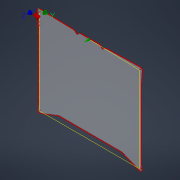
# Autodesk Inventor part: left_plate_02
Saved by Autodesk Inventor 2022 (Build 260153000, 153)
## iProperties
Created: 2025-02-08
Part Number: left_plate_02
Material: ポリカーボネート、クリア
Document SubType Name: Modeling
Designer: gisen
Density: 1.2 g/cm^3
Appearance: ポリカーボネート - クリア
Mass: 702.693 g
Surface Area: 3961.4 cm^2
Volume: 585.578 cm^3
Author: gisen
Autodesk Inventor part; units mm, degrees
ref_plane "YZ Plane" through (0, 0, 0) normal (1, 0, 0) x (0, 1, 0)
ref_plane "XZ Plane" through (0, 0, 0) normal (0, 1, 0) x (-1, 0, 0)
ref_plane "XY Plane" through (0, 0, 0) normal (0, 0, 1) x (1, 0, 0)
sketch "スケッチ1" plane through (0, 0, 0) normal (0, 0, 1) x (1, 0, 0)
  circle A0 centre (-239, 204) radius 2.1 construction
  circle A1 centre (-239, -204) radius 2.1 construction
  circle A2 centre (239, -204) radius 2.1 construction
  circle A3 centre (239, 204) radius 2.1 construction
  circle A4 centre (-61, 204) radius 2.1 construction
  circle A5 centre (61, 204) radius 2.1 construction
  circle A6 centre (-50, -185) radius 2.1 construction
  circle A7 centre (-161.1336, -215) radius 2.1 construction
  circle A8 centre (50, -185) radius 2.1 construction
  circle A9 centre (150, -185) radius 2.1 construction
  circle A10 centre (161.1336, -215) radius 2.1 construction
  circle A11 centre (250, -185) radius 1.6 construction
  circle A12 centre (250, -215) radius 1.6 construction
  line L0 (239, 184) -> (239, -154) construction
  arc A13 (239, 184) -> (219, 204) centre (219, 184) ccw construction
  arc A14 (219, -174) -> (239, -154) centre (219, -154) ccw construction
  line L1 (219, -174) -> (-219, -174) construction
  line L2 (81, 204) -> (219, 204) construction
  line L3 (-239, -154) -> (-239, 184) construction
  arc A15 (-239, -154) -> (-219, -174) centre (-219, -154) ccw construction
  arc A16 (-219, 204) -> (-239, 184) centre (-219, 184) ccw construction
  line L4 (-219, 204) -> (-81, 204) construction
  arc A17 (-66.8579, 198.1421) -> (-55.1421, 198.1421) centre (-61, 204) ccw construction
  arc A18 (-66.8579, 198.1421) -> (-81, 204) centre (-81, 184) ccw construction
  arc A19 (-41, 204) -> (-55.1421, 198.1421) centre (-41, 184) ccw construction
  line L5 (-41, 204) -> (41, 204) construction
  arc A20 (55.1421, 198.1421) -> (41, 204) centre (41, 184) ccw construction
  arc A21 (55.1421, 198.1421) -> (66.8579, 198.1421) centre (61, 204) ccw construction
  arc A22 (81, 204) -> (66.8579, 198.1421) centre (81, 184) ccw construction
  circle A23 centre (-250, -215) radius 2.1 construction
  circle A24 centre (-239, 204) radius 10 construction
  circle A25 centre (-250, 215) radius 1.6 construction
  circle A26 centre (-250, 215) radius 5 construction
  circle A27 centre (-239, -204) radius 10 construction
  circle A28 centre (239, -204) radius 10 construction
  circle A29 centre (239, 204) radius 10 construction
  line L6 (245, -154) -> (245, 184) construction
  arc A30 (245, 184) -> (219, 210) centre (219, 184) ccw construction
  line L7 (219, 210) -> (81, 210) construction
  arc A31 (81, 210) -> (62.6152, 202.3848) centre (81, 184) ccw construction
  arc A32 (59.3848, 202.3848) -> (62.6152, 202.3848) centre (61, 204) ccw construction
  arc A33 (59.3848, 202.3848) -> (41, 210) centre (41, 184) ccw construction
  line L8 (41, 210) -> (-41, 210) construction
  arc A34 (-41, 210) -> (-59.3848, 202.3848) centre (-41, 184) ccw construction
  arc A35 (-62.6152, 202.3848) -> (-59.3848, 202.3848) centre (-61, 204) ccw construction
  arc A36 (-62.6152, 202.3848) -> (-81, 210) centre (-81, 184) ccw construction
  line L9 (-81, 210) -> (-219, 210) construction
  arc A37 (-219, 210) -> (-245, 184) centre (-219, 184) ccw construction
  line L10 (-245, 184) -> (-245, -154) construction
  arc A38 (-245, -154) -> (-219, -180) centre (-219, -154) ccw construction
  line L11 (-219, -180) -> (219, -180) construction
  arc A39 (219, -180) -> (245, -154) centre (219, -154) ccw construction
  circle A40 centre (250, -185) radius 5 construction
  circle A41 centre (250, 145) radius 2.1 construction
  circle A42 centre (250, 145) radius 5 construction
  circle A43 centre (150, -185) radius 5 construction
  circle A44 centre (61, 204) radius 5 construction
  line L12 (150.951, -180) -> (235.3288, -213.3018)
  line L13 (245, -154) -> (245, -185.5709)
  line L14 (245, -185.5709) -> (248.7426, -201.7457)
  arc A45 (235.3288, -213.3018) -> (248.7426, -201.7457) centre (239, -204) ccw
  line L15 (0, -174) -> (0, 204) construction
  line L16 (245, 145.1708) -> (248.9767, 203.3177)
  line L17 (238.7472, 213.9968) -> (80.3428, 209.9917)
  arc A46 (80.3428, 209.9917) -> (65.2441, 201.3566) centre (80.8062, 191.6636) ccw
  arc A47 (56.7774, 201.3225) -> (41, 210) centre (41, 191.3182) ccw
  arc A48 (56.7774, 201.3225) -> (65.2441, 201.3566) centre (61, 204) ccw
  line L18 (245, -154) -> (245, 145.1708)
  arc A49 (248.9767, 203.3177) -> (238.7472, 213.9968) centre (239, 204) ccw
  line L19 (-150.951, -180) -> (-235.3288, -213.3018)
  line L20 (-245, -154) -> (-245, -185.5709)
  line L21 (-245, -185.5709) -> (-248.7426, -201.7457)
  arc A50 (-248.7426, -201.7457) -> (-235.3288, -213.3018) centre (-239, -204) ccw
  line L22 (-245, 145.1708) -> (-248.9767, 203.3177)
  line L23 (-238.7472, 213.9968) -> (-80.3428, 209.9917)
  arc A51 (-65.2441, 201.3566) -> (-80.3428, 209.9917) centre (-80.8062, 191.6636) ccw
  arc A52 (-41, 210) -> (-56.7774, 201.3225) centre (-41, 191.3182) ccw
  arc A53 (-65.2441, 201.3566) -> (-56.7774, 201.3225) centre (-61, 204) ccw
  line L24 (-245, -154) -> (-245, 145.1708)
  arc A54 (-238.7472, 213.9968) -> (-248.9767, 203.3177) centre (-239, 204) ccw
  line L25 (-150.951, -180) -> (150.951, -180)
  line L26 (-41, 210) -> (41, 210)
  circle A55 centre (-239, -204) radius 2.1
  circle A56 centre (-239, 204) radius 2.1
  circle A57 centre (239, 204) radius 2.1
  circle A58 centre (239, -204) radius 2.1
  point P0 (0, 0)
  dimension "d0" = 20
  dimension "d1" = 10
  dimension "d2" = 6
  dimension "d3" = 10
  dimension "d4" = 4.2
  constraints: 47 point on circle, 42 end point, 33 centre point, 16 coincident, 15 symmetric about line, 13 tangent, 9 equal radius, 3 collinear, 2 midpoint, 2 point on line, 1 vertical, 20 other
  measures "d0" diameter of A24
  measures "d1" diameter of A26
  measures "d2" radial gap between concentric circles of A14 A39
  measures "d3" diameter of A40
  measures "d4" diameter of A55
extrude "押し出し1" add sketch "スケッチ1" along normal blind 3
sketch "スケッチ2" plane through (0, 0, 3) normal (0, 0, 1) x (1, 0, 0)
  circle A0 centre (-250, -200) radius 2.1 construction
  circle A1 centre (-250, -200) radius 5
  line L0 (41, 210) -> (-41, 210) construction
  line L1 (-150.951, -180) -> (150.951, -180) construction
  line L2 (0, 210) -> (0, -180) construction
  circle A2 centre (250, -200) radius 5
  point P0 (0, 0)
  dimension "d7" = 10
  constraints: 2 centre point, 2 end point, 2 midpoint, 1 coincident, 1 symmetric about line, 1 other
  measures "d7" diameter of A1
extrude "押し出し2" cut sketch "スケッチ2" against normal through all
fillet "フィレット1" radius 5 10 edges at (248.9603, -204.8907, 1.5) (247.3566, -195.7559, 1.5) (245, -185.5709, 1.5) (150.951, -180, 1.5) (245, 145.1708, 1.5) (-245, 145.1708, 1.5) (-245, -185.5709, 1.5) (-247.3566, -195.7559, 1.5) (-248.9603, -204.8907, 1.5) (-150.951, -180, 1.5)
